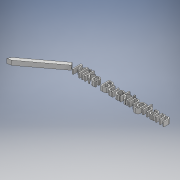
# Autodesk Inventor part: Mike2
Saved by Autodesk Inventor 2017 (Build 210142000, 142)
## iProperties
Created: 2021-02-26
Part Number: Mike2
Material: Generic
Document SubType Name: Modeling
Designer: paulg
Density: 1 g/cm^3
Appearance: Default
Author: paulg
Autodesk Inventor part; units mm, degrees
ref_plane "YZ Plane" through (0, 0, 0) normal (1, 0, 0) x (0, 1, 0)
ref_plane "XZ Plane" through (0, 0, 0) normal (0, 1, 0) x (-1, 0, 0)
ref_plane "XY Plane" through (0, 0, 0) normal (0, 0, 1) x (1, 0, 0)
sketch "Sketch1" plane through (0, 0, 0) normal (0, 0, 1) x (1, 0, 0)
  line L0 (-0.0217, 0.1086) -> (142.61, 0.1086) construction
  line L1 (142.61, 0.1086) -> (142.61, -1.7562) construction
  line L2 (142.61, -1.7562) -> (-0.0217, -1.7562) construction
  line L3 (-0.0217, -1.7562) -> (-0.0217, 0.1086) construction
  line L4 (-41.7116, -36.1087) -> (-2.9577, -7.16)
  line L5 (-2.9577, -7.16) -> (-5.3043, -4.0186)
  line L6 (-5.3043, -4.0186) -> (-44.0582, -32.9673)
  line L7 (-44.0582, -32.9673) -> (-41.7116, -36.1087)
  line L8 (-41.7116, -36.1087) -> (-5.3043, -4.0186) construction
  line L9 (-2.9577, -7.16) -> (-44.0582, -32.9673) construction
  line L10 (-44.0582, -32.9673) -> (-46.1916, -37.008)
  line L11 (-46.1916, -37.008) -> (-41.7116, -36.1087)
  line L12 (-46.1916, -37.008) -> (-42.8849, -34.538) construction
  line L13 (9.565, -10.3371) -> (8.236, -10.3371)
  line L14 (8.236, -10.3371) -> (8.236, -1.7228)
  line L15 (8.236, -1.7228) -> (5.6266, -7.5818)
  line L16 (5.6266, -7.5818) -> (4.8162, -7.5818)
  line L17 (4.8162, -7.5818) -> (2.2311, -1.7228)
  line L18 (2.2311, -1.7228) -> (2.2311, -10.3371)
  line L19 (2.2311, -10.3371) -> (0.9912, -10.3371)
  line L20 (0.9912, -10.3371) -> (0.9912, -0.3371)
  line L21 (0.9912, -0.3371) -> (2.8065, -0.3371)
  line L22 (2.8065, -0.3371) -> (5.3024, -5.9043)
  line L23 (5.3024, -5.9043) -> (7.7173, -0.3371)
  line L24 (7.7173, -0.3371) -> (9.565, -0.3371)
  line L25 (9.565, -0.3371) -> (9.565, -10.3371)
  line L26 (12.7822, -10.3371) -> (11.518, -10.3371)
  line L27 (11.518, -10.3371) -> (11.518, -2.833)
  line L28 (11.518, -2.833) -> (12.7822, -2.833)
  line L29 (12.7822, -2.833) -> (12.7822, -10.3371)
  line L30 (12.8713, -1.585) -> (11.4369, -1.585)
  line L31 (11.4369, -1.585) -> (11.4369, -0.2722)
  line L32 (11.4369, -0.2722) -> (12.8713, -0.2722)
  line L33 (12.8713, -0.2722) -> (12.8713, -1.585)
  line L34 (20.8535, -10.3371) -> (19.1922, -10.3371)
  line L35 (19.1922, -10.3371) -> (16.4045, -6.7147)
  line L36 (16.4045, -6.7147) -> (15.9021, -7.2009)
  line L37 (15.9021, -7.2009) -> (15.9021, -10.3371)
  line L38 (15.9021, -10.3371) -> (14.6379, -10.3371)
  line L39 (14.6379, -10.3371) -> (14.6379, 0.1086)
  line L40 (14.6379, 0.1086) -> (15.9021, 0.1086)
  line L41 (15.9021, 0.1086) -> (15.9021, -6.0016)
  line L42 (15.9021, -6.0016) -> (18.8681, -2.833)
  line L43 (18.8681, -2.833) -> (20.4402, -2.833)
  line L44 (20.4402, -2.833) -> (17.3608, -5.9692)
  line L45 (17.3608, -5.9692) -> (20.8535, -10.3371)
  spline S0 degree 2 poles (24.7433, -10.5072) (22.9442, -10.5072) (20.9669, -8.4894) (20.9669, -6.6256) knots 0 0 0 1 2 2 2
  spline S1 degree 2 poles (20.9669, -6.6256) (20.9669, -4.7941) (22.8875, -2.6223) (24.4353, -2.6223) knots 0 0 0 1 2 2 2
  spline S2 degree 2 poles (24.4353, -2.6223) (25.1322, -2.6223) (26.21, -3.0275) (26.6071, -3.457) knots 0 0 0 1 2 2 2
  spline S3 degree 2 poles (26.6071, -3.457) (27.0123, -3.8865) (27.4418, -5.1264) (27.4418, -6.0259) knots 0 0 0 1 2 2 2
  line L46 (27.4418, -6.0259) -> (27.4418, -6.7147)
  line L47 (27.4418, -6.7147) -> (22.2473, -6.7147)
  spline S4 degree 2 poles (22.2473, -6.7147) (22.2473, -8.0194) (23.5601, -9.4051) (24.7271, -9.4051) knots 0 0 0 1 2 2 2
  spline S5 degree 2 poles (24.7271, -9.4051) (25.1403, -9.4051) (25.9426, -9.2187) (26.2668, -9.0729) knots 0 0 0 1 2 2 2
  spline S6 degree 2 poles (26.2668, -9.0729) (26.6071, -8.9108) (27.0771, -8.6272) (27.2311, -8.4975) knots 0 0 0 1 2 2 2
  line L48 (27.2311, -8.4975) -> (27.304, -8.4975)
  line L49 (27.304, -8.4975) -> (27.304, -9.8751)
  spline S7 degree 2 poles (27.304, -9.8751) (27.0852, -9.9643) (26.4207, -10.2236) (26.1614, -10.2965) knots 0 0 0 1 2 2 2
  spline S8 degree 2 poles (26.1614, -10.2965) (25.7967, -10.4019) (25.1971, -10.5072) (24.7433, -10.5072) knots 0 0 0 1 2 2 2
  spline S9 degree 2 poles (26.21, -5.7503) (26.1938, -5.2398) (25.9831, -4.4943) (25.7805, -4.2431) knots 0 0 0 1 2 2 2
  spline S10 degree 2 poles (25.7805, -4.2431) (25.5617, -3.9594) (24.8729, -3.6596) (24.3624, -3.6596) knots 0 0 0 1 2 2 2
  spline S11 degree 2 poles (24.3624, -3.6596) (23.86, -3.6596) (23.1549, -3.9594) (22.8632, -4.2512) knots 0 0 0 1 2 2 2
  spline S12 degree 2 poles (22.8632, -4.2512) (22.5796, -4.551) (22.2878, -5.2722) (22.2473, -5.7503) knots 0 0 0 1 2 2 2
  line L50 (22.2473, -5.7503) -> (26.21, -5.7503)
  spline S13 degree 2 poles (39.8972, -7.2657) (39.8972, -8.0113) (39.33, -9.1539) (38.86, -9.5267) knots 0 0 0 1 2 2 2
  spline S14 degree 2 poles (38.86, -9.5267) (38.2927, -9.9643) (37.0042, -10.3371) (35.9831, -10.3371) knots 0 0 0 1 2 2 2
  line L51 (35.9831, -10.3371) -> (33.1144, -10.3371)
  line L52 (33.1144, -10.3371) -> (33.1144, -0.3371)
  line L53 (33.1144, -0.3371) -> (35.7643, -0.3371)
  spline S15 degree 2 poles (35.7643, -0.3371) (36.834, -0.3371) (37.9037, -0.4748) (38.3899, -0.7422) knots 0 0 0 1 2 2 2
  spline S16 degree 2 poles (38.3899, -0.7422) (38.9329, -1.0259) (39.4272, -1.9578) (39.4272, -2.5899) knots 0 0 0 1 2 2 2
  spline S17 degree 2 poles (39.4272, -2.5899) (39.4272, -3.2949) (38.6817, -4.4132) (38.0253, -4.7293) knots 0 0 0 1 2 2 2
  line L54 (38.0253, -4.7293) -> (38.0253, -4.7779)
  spline S18 degree 2 poles (38.0253, -4.7779) (38.9167, -5.021) (39.8972, -6.3095) (39.8972, -7.2657) knots 0 0 0 1 2 2 2
  spline S19 degree 2 poles (38.5115, -7.3225) (38.5115, -6.7552) (38.1873, -6.0259) (37.7011, -5.7666) knots 0 0 0 1 2 2 2
  spline S20 degree 2 poles (37.7011, -5.7666) (37.3851, -5.6045) (36.6395, -5.5072) (35.9507, -5.5072) knots 0 0 0 1 2 2 2
  line L55 (35.9507, -5.5072) -> (34.4434, -5.5072)
  line L56 (34.4434, -5.5072) -> (34.4434, -9.2025)
  line L57 (34.4434, -9.2025) -> (35.5212, -9.2025)
  spline S21 degree 2 poles (35.5212, -9.2025) (36.3964, -9.2025) (37.4013, -9.0405) (37.7903, -8.7811) knots 0 0 0 1 2 2 2
  spline S22 degree 2 poles (37.7903, -8.7811) (38.163, -8.5137) (38.5115, -7.8492) (38.5115, -7.3225) knots 0 0 0 1 2 2 2
  spline S23 degree 2 poles (38.0415, -2.7763) (38.0415, -2.4197) (37.7984, -1.8849) (37.5309, -1.7309) knots 0 0 0 1 2 2 2
  spline S24 degree 2 poles (37.5309, -1.7309) (37.2068, -1.5526) (36.4207, -1.4716) (35.7157, -1.4716) knots 0 0 0 1 2 2 2
  line L58 (35.7157, -1.4716) -> (34.4434, -1.4716)
  line L59 (34.4434, -1.4716) -> (34.4434, -4.397)
  line L60 (34.4434, -4.397) -> (35.9507, -4.397)
  spline S25 degree 2 poles (35.9507, -4.397) (36.5747, -4.397) (37.1663, -4.2674) (37.4823, -4.0648) knots 0 0 0 1 2 2 2
  spline S26 degree 2 poles (37.4823, -4.0648) (37.7903, -3.8703) (38.0415, -3.2463) (38.0415, -2.7763) knots 0 0 0 1 2 2 2
  line L61 (46.9556, -10.3371) -> (45.6914, -10.3371)
  line L62 (45.6914, -10.3371) -> (45.6914, -9.5105)
  spline S27 degree 2 poles (45.6914, -9.5105) (45.1079, -10.021) (44.0625, -10.5478) (43.4143, -10.5478) knots 0 0 0 1 2 2 2
  spline S28 degree 2 poles (43.4143, -10.5478) (42.928, -10.5478) (42.0609, -10.2236) (41.7449, -9.8751) knots 0 0 0 1 2 2 2
  spline S29 degree 2 poles (41.7449, -9.8751) (41.4207, -9.5267) (41.0642, -8.4651) (41.0642, -7.7033) knots 0 0 0 1 2 2 2
  line L63 (41.0642, -7.7033) -> (41.0642, -2.833)
  line L64 (41.0642, -2.833) -> (42.3284, -2.833)
  line L65 (42.3284, -2.833) -> (42.3284, -7.1118)
  spline S30 degree 2 poles (42.3284, -7.1118) (42.3284, -7.7115) (42.4175, -8.4975) (42.5715, -8.7892) knots 0 0 0 1 2 2 2
  spline S31 degree 2 poles (42.5715, -8.7892) (42.7254, -9.081) (43.2522, -9.3484) (43.7465, -9.3484) knots 0 0 0 1 2 2 2
  spline S32 degree 2 poles (43.7465, -9.3484) (44.2084, -9.3484) (45.2538, -8.8217) (45.6914, -8.4408) knots 0 0 0 1 2 2 2
  line L66 (45.6914, -8.4408) -> (45.6914, -2.833)
  line L67 (45.6914, -2.833) -> (46.9556, -2.833)
  line L68 (46.9556, -2.833) -> (46.9556, -10.3371)
  spline S33 degree 2 poles (51.7692, -10.5072) (50.9912, -10.5072) (49.7027, -10.0291) (49.2408, -9.5429) knots 0 0 0 1 2 2 2
  spline S34 degree 2 poles (49.2408, -9.5429) (48.7789, -9.0648) (48.2684, -7.5899) (48.2684, -6.6012) knots 0 0 0 1 2 2 2
  spline S35 degree 2 poles (48.2684, -6.6012) (48.2684, -5.6126) (48.7951, -4.1701) (49.2408, -3.6839) knots 0 0 0 1 2 2 2
  spline S36 degree 2 poles (49.2408, -3.6839) (49.6865, -3.1896) (51.0074, -2.6628) (51.7692, -2.6628) knots 0 0 0 1 2 2 2
  spline S37 degree 2 poles (51.7692, -2.6628) (52.3851, -2.6628) (53.5358, -3.0113) (53.9815, -3.2382) knots 0 0 0 1 2 2 2
  line L69 (53.9815, -3.2382) -> (53.9815, -4.6563)
  line L70 (53.9815, -4.6563) -> (53.9086, -4.6563)
  spline S38 degree 2 poles (53.9086, -4.6563) (53.7708, -4.5429) (53.3494, -4.2512) (53.0496, -4.0972) knots 0 0 0 1 2 2 2
  spline S39 degree 2 poles (53.0496, -4.0972) (52.7822, -3.9675) (52.069, -3.7649) (51.7449, -3.7649) knots 0 0 0 1 2 2 2
  spline S40 degree 2 poles (51.7449, -3.7649) (50.7643, -3.7649) (49.5731, -5.2479) (49.5731, -6.6012) knots 0 0 0 1 2 2 2
  spline S41 degree 2 poles (49.5731, -6.6012) (49.5731, -7.9221) (50.7238, -9.4051) (51.7449, -9.4051) knots 0 0 0 1 2 2 2
  spline S42 degree 2 poles (51.7449, -9.4051) (52.3608, -9.4051) (53.4791, -8.8946) (53.9086, -8.4975) knots 0 0 0 1 2 2 2
  line L71 (53.9086, -8.4975) -> (53.9815, -8.4975)
  line L72 (53.9815, -8.4975) -> (53.9815, -9.9157)
  spline S43 degree 2 poles (53.9815, -9.9157) (53.7951, -10.0048) (53.2279, -10.256) (53.001, -10.3127) knots 0 0 0 1 2 2 2
  spline S44 degree 2 poles (53.001, -10.3127) (52.6768, -10.41) (52.1663, -10.5072) (51.7692, -10.5072) knots 0 0 0 1 2 2 2
  line L73 (61.3478, -10.3371) -> (59.6865, -10.3371)
  line L74 (59.6865, -10.3371) -> (56.8989, -6.7147)
  line L75 (56.8989, -6.7147) -> (56.3964, -7.2009)
  line L76 (56.3964, -7.2009) -> (56.3964, -10.3371)
  line L77 (56.3964, -10.3371) -> (55.1322, -10.3371)
  line L78 (55.1322, -10.3371) -> (55.1322, 0.1086)
  line L79 (55.1322, 0.1086) -> (56.3964, 0.1086)
  line L80 (56.3964, 0.1086) -> (56.3964, -6.0016)
  line L81 (56.3964, -6.0016) -> (59.3624, -2.833)
  line L82 (59.3624, -2.833) -> (60.9345, -2.833)
  line L83 (60.9345, -2.833) -> (57.8551, -5.9692)
  line L84 (57.8551, -5.9692) -> (61.3478, -10.3371)
  line L85 (63.2684, -10.3371) -> (62.0042, -10.3371)
  line L86 (62.0042, -10.3371) -> (62.0042, -2.833)
  line L87 (62.0042, -2.833) -> (63.2684, -2.833)
  line L88 (63.2684, -2.833) -> (63.2684, -10.3371)
  line L89 (63.3575, -1.585) -> (61.9232, -1.585)
  line L90 (61.9232, -1.585) -> (61.9232, -0.2722)
  line L91 (61.9232, -0.2722) -> (63.3575, -0.2722)
  line L92 (63.3575, -0.2722) -> (63.3575, -1.585)
  line L93 (71.0155, -10.3371) -> (69.7514, -10.3371)
  line L94 (69.7514, -10.3371) -> (69.7514, -6.0583)
  spline S45 degree 2 poles (69.7514, -6.0583) (69.7514, -5.5397) (69.6541, -4.6482) (69.5083, -4.3808) knots 0 0 0 1 2 2 2
  spline S46 degree 2 poles (69.5083, -4.3808) (69.3543, -4.0972) (68.8032, -3.8217) (68.3332, -3.8217) knots 0 0 0 1 2 2 2
  spline S47 degree 2 poles (68.3332, -3.8217) (67.8632, -3.8217) (66.8664, -4.3241) (66.3883, -4.7293) knots 0 0 0 1 2 2 2
  line L95 (66.3883, -4.7293) -> (66.3883, -10.3371)
  line L96 (66.3883, -10.3371) -> (65.1241, -10.3371)
  line L97 (65.1241, -10.3371) -> (65.1241, -2.833)
  line L98 (65.1241, -2.833) -> (66.3883, -2.833)
  line L99 (66.3883, -2.833) -> (66.3883, -3.6677)
  spline S48 degree 2 poles (66.3883, -3.6677) (66.9556, -3.1572) (68.0496, -2.6223) (68.6655, -2.6223) knots 0 0 0 1 2 2 2
  spline S49 degree 2 poles (68.6655, -2.6223) (69.7676, -2.6223) (71.0155, -4.081) (71.0155, -5.4667) knots 0 0 0 1 2 2 2
  line L100 (71.0155, -5.4667) -> (71.0155, -10.3371)
  spline S50 degree 2 poles (73.0577, -11.5364) (73.1873, -11.5931) (73.6817, -11.7714) (73.9977, -11.8444) knots 0 0 0 1 2 2 2
  spline S51 degree 2 poles (73.9977, -11.8444) (74.3462, -11.9335) (74.9378, -12.0388) (75.2862, -12.0388) knots 0 0 0 1 2 2 2
  spline S52 degree 2 poles (75.2862, -12.0388) (75.8697, -12.0388) (76.6801, -11.7309) (76.907, -11.4554) knots 0 0 0 1 2 2 2
  spline S53 degree 2 poles (76.907, -11.4554) (77.1258, -11.1798) (77.2959, -10.4586) (77.2959, -9.9967) knots 0 0 0 1 2 2 2
  line L101 (77.2959, -9.9967) -> (77.2959, -9.3403)
  spline S54 degree 2 poles (77.2959, -9.3403) (76.7854, -9.786) (75.8049, -10.2074) (75.0674, -10.2074) knots 0 0 0 1 2 2 2
  spline S55 degree 2 poles (75.0674, -10.2074) (73.787, -10.2074) (72.2716, -8.303) (72.2716, -6.5121) knots 0 0 0 1 2 2 2
  spline S56 degree 2 poles (72.2716, -6.5121) (72.2716, -5.5802) (72.7984, -4.1377) (73.236, -3.6272) knots 0 0 0 1 2 2 2
  spline S57 degree 2 poles (73.236, -3.6272) (73.6574, -3.1491) (74.8162, -2.6223) (75.4321, -2.6223) knots 0 0 0 1 2 2 2
  spline S58 degree 2 poles (75.4321, -2.6223) (76.0155, -2.6223) (76.8664, -2.8978) (77.2959, -3.1491) knots 0 0 0 1 2 2 2
  line L102 (77.2959, -3.1491) -> (77.3689, -2.833)
  line L103 (77.3689, -2.833) -> (78.5601, -2.833)
  line L104 (78.5601, -2.833) -> (78.5601, -9.4781)
  spline S59 degree 2 poles (78.5601, -9.4781) (78.5601, -11.3905) (76.8989, -13.1734) (75.189, -13.1734) knots 0 0 0 1 2 2 2
  spline S60 degree 2 poles (75.189, -13.1734) (74.6379, -13.1734) (73.4872, -12.9951) (72.9929, -12.8492) knots 0 0 0 1 2 2 2
  line L105 (72.9929, -12.8492) -> (72.9929, -11.5364)
  line L106 (72.9929, -11.5364) -> (73.0577, -11.5364)
  line L107 (77.2959, -8.303) -> (77.2959, -4.1782)
  spline S61 degree 2 poles (77.2959, -4.1782) (76.8259, -3.9513) (76.0318, -3.7568) (75.6347, -3.7568) knots 0 0 0 1 2 2 2
  spline S62 degree 2 poles (75.6347, -3.7568) (74.6784, -3.7568) (73.5763, -5.1669) (73.5763, -6.4878) knots 0 0 0 1 2 2 2
  spline S63 degree 2 poles (73.5763, -6.4878) (73.5763, -7.7358) (74.411, -9.0405) (75.351, -9.0405) knots 0 0 0 1 2 2 2
  spline S64 degree 2 poles (75.351, -9.0405) (75.8454, -9.0405) (76.8826, -8.6515) (77.2959, -8.303) knots 0 0 0 1 2 2 2
  line L108 (86.283, -10.3371) -> (85.0188, -10.3371)
  line L109 (85.0188, -10.3371) -> (85.0188, -6.0583)
  spline S65 degree 2 poles (85.0188, -6.0583) (85.0188, -5.5397) (84.9215, -4.6482) (84.7757, -4.3808) knots 0 0 0 1 2 2 2
  spline S66 degree 2 poles (84.7757, -4.3808) (84.6217, -4.0972) (84.0707, -3.8217) (83.6006, -3.8217) knots 0 0 0 1 2 2 2
  spline S67 degree 2 poles (83.6006, -3.8217) (83.1306, -3.8217) (82.1339, -4.3241) (81.6557, -4.7293) knots 0 0 0 1 2 2 2
  line L110 (81.6557, -4.7293) -> (81.6557, -10.3371)
  line L111 (81.6557, -10.3371) -> (80.3916, -10.3371)
  line L112 (80.3916, -10.3371) -> (80.3916, 0.1086)
  line L113 (80.3916, 0.1086) -> (81.6557, 0.1086)
  line L114 (81.6557, 0.1086) -> (81.6557, -3.6677)
  spline S68 degree 2 poles (81.6557, -3.6677) (82.223, -3.1572) (83.317, -2.6223) (83.9329, -2.6223) knots 0 0 0 1 2 2 2
  spline S69 degree 2 poles (83.9329, -2.6223) (85.035, -2.6223) (86.283, -4.081) (86.283, -5.4667) knots 0 0 0 1 2 2 2
  line L115 (86.283, -5.4667) -> (86.283, -10.3371)
  spline S70 degree 2 poles (92.2392, -9.5429) (92.0852, -9.6563) (91.5666, -10.0615) (91.3235, -10.1831) knots 0 0 0 1 2 2 2
  spline S71 degree 2 poles (91.3235, -10.1831) (90.9912, -10.3614) (90.3672, -10.5478) (89.8, -10.5478) knots 0 0 0 1 2 2 2
  spline S72 degree 2 poles (89.8, -10.5478) (89.3381, -10.5478) (88.5034, -10.1993) (88.1873, -9.8833) knots 0 0 0 1 2 2 2
  spline S73 degree 2 poles (88.1873, -9.8833) (87.8875, -9.5753) (87.5228, -8.6677) (87.5228, -8.1653) knots 0 0 0 1 2 2 2
  spline S74 degree 2 poles (87.5228, -8.1653) (87.5228, -7.3873) (88.1792, -6.2852) (88.8924, -5.9692) knots 0 0 0 1 2 2 2
  spline S75 degree 2 poles (88.8924, -5.9692) (89.5245, -5.6774) (91.2425, -5.4586) (92.2392, -5.4019) knots 0 0 0 1 2 2 2
  line L116 (92.2392, -5.4019) -> (92.2392, -5.1588)
  spline S76 degree 2 poles (92.2392, -5.1588) (92.2392, -4.7212) (91.9718, -4.1782) (91.7287, -4.0243) knots 0 0 0 1 2 2 2
  spline S77 degree 2 poles (91.7287, -4.0243) (91.4856, -3.8703) (90.7886, -3.773) (90.4159, -3.773) knots 0 0 0 1 2 2 2
  spline S78 degree 2 poles (90.4159, -3.773) (89.9783, -3.773) (88.7951, -4.0324) (88.2036, -4.2836) knots 0 0 0 1 2 2 2
  line L117 (88.2036, -4.2836) -> (88.1306, -4.2836)
  line L118 (88.1306, -4.2836) -> (88.1306, -2.9951)
  spline S79 degree 2 poles (88.1306, -2.9951) (88.4791, -2.8978) (89.7838, -2.6547) (90.424, -2.6547) knots 0 0 0 1 2 2 2
  spline S80 degree 2 poles (90.424, -2.6547) (91.2019, -2.6547) (92.2635, -2.8978) (92.6849, -3.2139) knots 0 0 0 1 2 2 2
  spline S81 degree 2 poles (92.6849, -3.2139) (93.0982, -3.5218) (93.5034, -4.5024) (93.5034, -5.2074) knots 0 0 0 1 2 2 2
  line L119 (93.5034, -5.2074) -> (93.5034, -10.3371)
  line L120 (93.5034, -10.3371) -> (92.2392, -10.3371)
  line L121 (92.2392, -10.3371) -> (92.2392, -9.5429)
  line L122 (92.2392, -8.4894) -> (92.2392, -6.4068)
  spline S82 degree 2 poles (92.2392, -6.4068) (91.7854, -6.4473) (90.4159, -6.585) (89.9864, -6.7147) knots 0 0 0 1 2 2 2
  spline S83 degree 2 poles (89.9864, -6.7147) (89.4839, -6.8687) (88.8275, -7.5089) (88.8275, -8.0761) knots 0 0 0 1 2 2 2
  spline S84 degree 2 poles (88.8275, -8.0761) (88.8275, -8.7244) (89.5569, -9.3808) (90.2538, -9.3808) knots 0 0 0 1 2 2 2
  spline S85 degree 2 poles (90.2538, -9.3808) (90.8454, -9.3808) (91.8178, -8.8703) (92.2392, -8.4894) knots 0 0 0 1 2 2 2
  line L123 (103.787, -10.3371) -> (103.787, -5.9935)
  spline S86 degree 2 poles (103.787, -5.9935) (103.787, -5.4748) (103.706, -4.5915) (103.5763, -4.3484) knots 0 0 0 1 2 2 2
  spline S87 degree 2 poles (103.5763, -4.3484) (103.4467, -4.081) (102.9523, -3.8217) (102.5228, -3.8217) knots 0 0 0 1 2 2 2
  spline S88 degree 2 poles (102.5228, -3.8217) (102.1339, -3.8217) (101.2425, -4.2998) (100.7724, -4.7536) knots 0 0 0 1 2 2 2
  spline S89 degree 2 poles (100.7724, -4.7536) (100.7805, -4.867) (100.7967, -5.1831) (100.7967, -5.3938) knots 0 0 0 1 2 2 2
  line L124 (100.7967, -5.3938) -> (100.7967, -10.3371)
  line L125 (100.7967, -10.3371) -> (99.5326, -10.3371)
  line L126 (99.5326, -10.3371) -> (99.5326, -5.9935)
  spline S90 degree 2 poles (99.5326, -5.9935) (99.5326, -5.4748) (99.4515, -4.5915) (99.3219, -4.3484) knots 0 0 0 1 2 2 2
  spline S91 degree 2 poles (99.3219, -4.3484) (99.1922, -4.081) (98.6979, -3.8217) (98.2684, -3.8217) knots 0 0 0 1 2 2 2
  spline S92 degree 2 poles (98.2684, -3.8217) (97.8632, -3.8217) (96.9637, -4.3322) (96.5423, -4.7293) knots 0 0 0 1 2 2 2
  line L127 (96.5423, -4.7293) -> (96.5423, -10.3371)
  line L128 (96.5423, -10.3371) -> (95.2781, -10.3371)
  line L129 (95.2781, -10.3371) -> (95.2781, -2.833)
  line L130 (95.2781, -2.833) -> (96.5423, -2.833)
  line L131 (96.5423, -2.833) -> (96.5423, -3.6596)
  spline S93 degree 2 poles (96.5423, -3.6596) (97.0366, -3.1653) (98.0091, -2.6223) (98.5925, -2.6223) knots 0 0 0 1 2 2 2
  spline S94 degree 2 poles (98.5925, -2.6223) (99.257, -2.6223) (100.2862, -3.2301) (100.5536, -3.9189) knots 0 0 0 1 2 2 2
  spline S95 degree 2 poles (100.5536, -3.9189) (101.129, -3.2787) (102.2149, -2.6223) (102.847, -2.6223) knots 0 0 0 1 2 2 2
  spline S96 degree 2 poles (102.847, -2.6223) (103.3332, -2.6223) (104.1274, -2.9221) (104.4191, -3.2625) knots 0 0 0 1 2 2 2
  spline S97 degree 2 poles (104.4191, -3.2625) (104.719, -3.6029) (105.0512, -4.6239) (105.0512, -5.3938) knots 0 0 0 1 2 2 2
  line L132 (105.0512, -5.3938) -> (105.0512, -10.3371)
  line L133 (105.0512, -10.3371) -> (103.787, -10.3371)
  point P0 (0, 0)
  point P1 (-23.5079, -20.0636)
  constraints: 18 end point, 3 midpoint, 3 parallel, 1 perpendicular, 2 other
extrude "Extrusion1" add sketch "Sketch1" along normal blind 5
body "Solid1"
